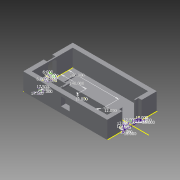
# Autodesk Inventor part: West_Structure_1st_Floor
Saved by Autodesk Inventor 2014 (Build 180170000, 170)
## iProperties
Created: 2013-07-10
Part Number: West_Structure_1st_Floor
Material: Generic
Document SubType Name: Modeling
Designer: jmw3
Density: 1 g/cm^3
Appearance: Default
Author: jmw3
Autodesk Inventor part; units mm, degrees
ref_plane "YZ Plane" through (0, 0, 0) normal (1, 0, 0) x (0, 1, 0)
ref_plane "XZ Plane" through (0, 0, 0) normal (0, 1, 0) x (-1, 0, 0)
ref_plane "XY Plane" through (0, 0, 0) normal (0, 0, 1) x (1, 0, 0)
sketch "Sketch1" plane through (0, 0, 0) normal (0, 0, 1) x (1, 0, 0)
  line L0 (-8321.04, 0) -> (8321.04, 0) projected
  line L1 (-5943.6, 3505.2) -> (5943.6, 3505.2)
  line L2 (-5334, 2895.6) -> (5334, 2895.6)
  line L3 (-4572, 2895.6) -> (-4419.6, 2895.6)
  line L4 (-1981.2, -2006.6) -> (-4445, -2006.6)
  line L5 (-4445, -2006.6) -> (-4445, -1892.3)
  line L6 (-1219.2, -2895.6) -> (-1066.8, -2895.6)
  line L7 (5334, -2895.6) -> (0, -2895.6)
  line L8 (0, -2895.6) -> (-5334, -2895.6)
  line L9 (5943.6, -3505.2) -> (0, -3505.2)
  line L10 (0, -3505.2) -> (-5943.6, -3505.2)
  line L11 (5334, 914.4) -> (5943.6, 914.4)
  line L12 (5943.6, -914.4) -> (5334, -914.4)
  line L13 (5334, 2895.6) -> (5334, 914.4)
  line L14 (5334, -914.4) -> (5334, -2895.6)
  line L15 (5943.6, 3505.2) -> (5943.6, 914.4)
  line L16 (5943.6, -914.4) -> (5943.6, -3505.2)
  line L17 (-4445, -2006.6) -> (5334, -2006.6)
  line L18 (5334, -1892.3) -> (-4445, -1892.3)
  line L19 (-4445, -1892.3) -> (-4445, -2006.6)
  line L20 (5334, -1892.3) -> (5334, -2006.6)
  line L21 (-5943.6, 609.6) -> (-5334, 609.6)
  line L22 (-5334, -609.6) -> (-5943.6, -609.6)
  line L23 (-5943.6, -3505.2) -> (-5943.6, -609.6)
  line L24 (-5943.6, 609.6) -> (-5943.6, 3505.2)
  line L25 (-5334, -2895.6) -> (-5334, -609.6)
  line L26 (-5334, 609.6) -> (-5334, 2895.6)
  line L27 (-4445, -2006.6) -> (-4419.6, -2006.6)
  line L28 (-4419.6, 2895.6) -> (-4572, 2895.6)
  line L29 (-4445, -1892.3) -> (-4445, -2006.6)
  line L30 (0, -4907.28) -> (0, 4907.28) projected
  dimension "d202" = 0
  dimension "d18" = 7010.4
  dimension "d19" = 609.6
  dimension "d20" = 609.6
  dimension "d23" = 1828.8
  dimension "d24" = 2590.8
  dimension "d25" = 609.6
  dimension "d28" = 114.3
  dimension "d29" = 0
  dimension "d34" = 1219.2
  dimension "d35" = 2895.6
  dimension "d36" = 609.6
  dimension "d46" = 889
  dimension "d105" = 889
  dimension "d106" = 11887.2
  constraints: 58 end point, 17 parallel, 8 horizontal, 7 collinear, 6 perpendicular, 4 point on line, 2 other
  measures "d18" distance between parallel lines of L10 L1
  measures "d19" distance between parallel lines of L10 L8
  measures "d20" distance between parallel lines of L1 L2
  measures "d23" distance between parallel lines of L12 L11
  measures "d24" distance between parallel lines of L9 L12
  measures "d25" distance between parallel lines of L15 L13
  measures "d28" distance between parallel lines of L17 L18
  measures "d29" distance between parallel lines of L13 L20
  measures "d34" distance between parallel lines of L22 L21
  measures "d35" distance between parallel lines of L10 L22
  measures "d36" distance between parallel lines of L24 L26
  measures "d46" distance between parallel lines of L26 L5
  measures "d105" distance from line of L6.end L17
  measures "d106" distance between parallel lines of L15 L24
extrude "Extrusion9" add sketch "Sketch1" along normal blind 2438.4 contours L18 L14 L17 L30 | L30 L17 L4 L5 L18 | L1 L30 L2 L26 L21 L24 | L1 L15 L11 L13 L2 L30 | L14 L12 L16 L9 L30 L7 | L30 L10 L23 L22 L25 L8 L6
sketch "Sketch8" plane through (0, 0, 0) normal (0, 0, -1) x (-1, 0, 0)
  line L0 (5943.6, 3505.2) -> (-5943.6, 3505.2) projected
  line L1 (-5943.6, 3505.2) -> (-5943.6, 914.4) projected
  line L2 (-5943.6, 914.4) -> (-5334, 914.4) projected
  line L3 (-5334, 914.4) -> (-5334, 2895.6) projected
  line L4 (-5334, 2895.6) -> (5334, 2895.6) projected
  line L5 (5334, 2895.6) -> (5334, 609.6) projected
  line L6 (5334, 609.6) -> (5943.6, 609.6) projected
  line L7 (5943.6, 609.6) -> (5943.6, 3505.2) projected
  line L8 (-5943.6, 3505.2) -> (5943.6, 3505.2)
  line L9 (5943.6, 3505.2) -> (5943.6, -3505.2)
  line L10 (5943.6, -3505.2) -> (-5943.6, -3505.2)
  line L11 (-5943.6, -3505.2) -> (-5943.6, 3505.2)
  point P0 (0, 0)
  constraints: 8 end point, 2 parallel, 1 horizontal, 1 perpendicular
extrude "Extrusion10" add sketch "Sketch8" along normal blind 25.4
sketch "Sketch9" plane through (0, 0, 2438.4) normal (0, 0, 1) x (1, 0, 0)
  line L0 (5943.6, 3505.2) -> (-5943.6, 3505.2) projected
  line L1 (-5943.6, 3505.2) -> (-5943.6, 609.6) projected
  line L2 (-5943.6, 609.6) -> (-5334, 609.6) projected
  line L3 (-5334, 609.6) -> (-5334, 2895.6) projected
  line L4 (-5334, 2895.6) -> (5334, 2895.6) projected
  line L5 (5334, 2895.6) -> (5334, 914.4) projected
  line L6 (5334, 914.4) -> (5943.6, 914.4) projected
  line L7 (5943.6, 914.4) -> (5943.6, 3505.2) projected
  line L8 (-5943.6, 609.6) -> (-5334, 609.6)
  line L9 (-5334, 609.6) -> (-5334, -609.6)
  line L10 (-5334, -609.6) -> (-5943.6, -609.6)
  line L11 (-5943.6, -609.6) -> (-5943.6, 609.6)
  line L12 (5334, 914.4) -> (5943.6, 914.4)
  line L13 (5943.6, 914.4) -> (5943.6, -914.4)
  line L14 (5943.6, -914.4) -> (5334, -914.4)
  line L15 (5334, -914.4) -> (5334, 914.4)
  point P0 (0, 0)
  constraints: 16 end point, 4 parallel, 2 horizontal, 2 perpendicular
extrude "Extrusion11" add sketch "Sketch9" against normal blind 406.4 contours L13 L14 L15 L6 | L2 L9 L10 L11
sketch "Sketch10" plane through (-4445, -2006.6, 2438.4) normal (0, -1, 0) x (1, 0, 0)
  line L0 (0, -2438.4) -> (9779, -2438.4) projected
  line L1 (0, -2438.4) -> (0, 0) projected
  line L2 (723.9, -2438.4) -> (914.4, -2438.4)
  line L3 (914.4, -2438.4) -> (914.4, -2254.25)
  line L4 (914.4, -2254.25) -> (723.9, -2254.25)
  line L5 (723.9, -2254.25) -> (723.9, -2438.4)
  line L6 (914.4, -2254.25) -> (1104.9, -2254.25)
  line L7 (1104.9, -2254.25) -> (1104.9, -2070.1)
  line L8 (1104.9, -2070.1) -> (914.4, -2070.1)
  line L9 (914.4, -2070.1) -> (914.4, -2254.25)
  line L10 (1104.9, -2070.1) -> (1295.4, -2070.1)
  line L11 (1295.4, -2070.1) -> (1295.4, -1885.95)
  line L12 (1295.4, -1885.95) -> (1104.9, -1885.95)
  line L13 (1104.9, -1885.95) -> (1104.9, -2070.1)
  line L14 (1295.4, -1885.95) -> (1485.9, -1885.95)
  line L15 (1485.9, -1885.95) -> (1485.9, -1701.8)
  line L16 (1485.9, -1701.8) -> (1295.4, -1701.8)
  line L17 (1295.4, -1701.8) -> (1295.4, -1885.95)
  line L18 (1485.9, -1701.8) -> (1676.4, -1701.8)
  line L19 (1676.4, -1701.8) -> (1676.4, -1517.65)
  line L20 (1676.4, -1517.65) -> (1485.9, -1517.65)
  line L21 (1485.9, -1517.65) -> (1485.9, -1701.8)
  line L22 (1676.4, -1517.65) -> (1866.9, -1517.65)
  line L23 (1866.9, -1517.65) -> (1866.9, -1333.5)
  line L24 (1866.9, -1333.5) -> (1676.4, -1333.5)
  line L25 (1676.4, -1333.5) -> (1676.4, -1517.65)
  line L26 (1866.9, -1333.5) -> (2057.4, -1333.5)
  line L27 (2057.4, -1333.5) -> (2057.4, -1149.35)
  line L28 (2057.4, -1149.35) -> (1866.9, -1149.35)
  line L29 (1866.9, -1149.35) -> (1866.9, -1333.5)
  line L30 (2438.4, -965.2) -> (2438.4, -781.05)
  line L31 (2247.9, -1149.35) -> (2247.9, -965.2)
  line L32 (2247.9, -965.2) -> (2438.4, -965.2)
  line L33 (2438.4, -781.05) -> (2247.9, -781.05)
  line L34 (2247.9, -781.05) -> (2247.9, -965.2)
  line L35 (2057.4, -1149.35) -> (2247.9, -1149.35)
  line L36 (2247.9, -965.2) -> (2057.4, -965.2)
  line L37 (2057.4, -965.2) -> (2057.4, -1149.35)
  line L38 (2628.9, -781.05) -> (2628.9, -596.9)
  line L39 (2438.4, -781.05) -> (2628.9, -781.05)
  line L40 (2628.9, -596.9) -> (2438.4, -596.9)
  line L41 (2438.4, -596.9) -> (2438.4, -781.05)
  line L42 (3200.4, -228.6) -> (3200.4, -44.45)
  line L43 (3200.4, 139.7) -> (3200.4, -44.45)
  line L44 (3200.4, -44.45) -> (3390.9, -44.45)
  line L45 (3390.9, 139.7) -> (3200.4, 139.7)
  line L46 (3009.9, -44.45) -> (3009.9, -228.6)
  line L47 (3009.9, -228.6) -> (3200.4, -228.6)
  line L48 (3200.4, -44.45) -> (3009.9, -44.45)
  line L49 (3390.9, -44.45) -> (3390.9, 139.7)
  line L50 (3009.9, -412.75) -> (3009.9, -228.6)
  line L51 (3009.9, -228.6) -> (2819.4, -228.6)
  line L52 (2819.4, -412.75) -> (3009.9, -412.75)
  line L53 (2819.4, -228.6) -> (2819.4, -412.75)
  line L54 (2819.4, -596.9) -> (2819.4, -412.75)
  line L55 (2819.4, -412.75) -> (2628.9, -412.75)
  line L56 (2628.9, -596.9) -> (2819.4, -596.9)
  line L57 (2628.9, -412.75) -> (2628.9, -596.9)
  line L58 (3390.9, 139.7) -> (3581.4, 139.7)
  line L59 (3581.4, 139.7) -> (3581.4, 323.85)
  line L60 (3581.4, 323.85) -> (3390.9, 323.85)
  line L61 (3390.9, 323.85) -> (3390.9, 139.7)
  point P0 (8445.5, -2438.4)
  point P1 (4445, -2438.4)
  dimension "d113" = 190.5
  dimension "d115" = 184.15
  dimension "d116" = 723.9
  dimension "d117" = 190.5
  dimension "d118" = 184.15
  dimension "d119" = 190.5
  dimension "d120" = 184.15
  dimension "d121" = 190.5
  dimension "d122" = 184.15
  dimension "d123" = 190.5
  dimension "d124" = 184.15
  dimension "d125" = 190.5
  dimension "d126" = 184.15
  dimension "d127" = 190.5
  dimension "d128" = 184.15
  dimension "d129" = 190.5
  dimension "d130" = 184.15
  dimension "d131" = 190.5
  dimension "d132" = 184.15
  dimension "d133" = 190.5
  dimension "d134" = 184.15
  dimension "d135" = 190.5
  dimension "d136" = 184.15
  dimension "d137" = 190.5
  dimension "d138" = 184.15
  dimension "d139" = 190.5
  dimension "d140" = 184.15
  dimension "d141" = 190.5
  dimension "d142" = 184.15
  dimension "d154" = 184.15
  dimension "d155" = 190.5
  constraints: 120 end point, 30 parallel, 15 horizontal, 15 perpendicular, 12 collinear, 1 point on line
  measures "d113" distance between parallel lines of L3 L5
  measures "d115" distance between parallel lines of L4 L0
  measures "d116" distance between parallel lines of L1 L5
  measures "d117" distance between parallel lines of L9 L7
  measures "d118" distance between parallel lines of L8 L6
  measures "d119" distance between parallel lines of L11 L13
  measures "d120" distance between parallel lines of L12 L10
  measures "d121" distance between parallel lines of L17 L15
  measures "d122" distance between parallel lines of L16 L14
  measures "d123" distance between parallel lines of L19 L21
  measures "d124" distance between parallel lines of L20 L18
  measures "d125" distance between parallel lines of L25 L23
  measures "d126" distance between parallel lines of L24 L22
  measures "d127" distance between parallel lines of L27 L29
  measures "d128" distance between parallel lines of L28 L26
  measures "d129" distance between parallel lines of L37 L31
  measures "d130" distance between parallel lines of L36 L35
  measures "d131" distance between parallel lines of L30 L34
  measures "d132" distance between parallel lines of L33 L32
  measures "d133" distance between parallel lines of L38 L41
  measures "d134" distance between parallel lines of L40 L39
  measures "d135" distance between parallel lines of L57 L54
  measures "d136" distance between parallel lines of L55 L56
  measures "d137" distance between parallel lines of L50 L53
  measures "d138" distance between parallel lines of L51 L52
  measures "d139" distance between parallel lines of L46 L42
  measures "d140" distance between parallel lines of L48 L47
  measures "d141" distance between parallel lines of L49 L43
  measures "d142" distance between parallel lines of L45 L44
  measures "d154" distance between parallel lines of L58 L60
  measures "d155" distance between parallel lines of L61 L59
extrude "Extrusion12" add sketch "Sketch10" along normal up to surface (889 mm away)
sketch "Sketch11" plane through (-5943.6, -3505.2, 2438.4) normal (0, -1, 0) x (1, 0, 0)
  line L0 (5334, -406.4) -> (6553.2, -406.4)
  line L1 (6553.2, -406.4) -> (6553.2, -1625.6)
  line L2 (6553.2, -1625.6) -> (5334, -1625.6)
  line L3 (5334, -1625.6) -> (5334, -406.4)
  line L4 (11277.6, -2438.4) -> (2413, -2438.4) projected
  line L5 (5943.6, -2956.56) -> (5943.6, 492.76) projected
  point P0 (5943.6, -2438.4)
  dimension "d145" = 1219.2
  dimension "d147" = 1219.2
  dimension "d148" = 812.8
  constraints: 8 end point, 2 parallel, 1 horizontal, 1 perpendicular, 1 other
  measures "d145" distance between parallel lines of L0 L2
  measures "d147" distance between parallel lines of L1 L3
  measures "d148" distance between parallel lines of L4 L2
extrude "Extrusion13" cut sketch "Sketch11" against normal up to surface (609.6 mm away)
sketch "Sketch14" plane through (0, 0, 2032) normal (0, 0, -1) x (-1, 0, 0)
  line L0 (-5334, -914.4) -> (-5334, 914.4) projected
  line L1 (-5943.6, 914.4) -> (-5943.6, -914.4) projected
  line L2 (-8321.04, 0) -> (8321.04, 0) projected
  line L3 (-5943.6, 12.7) -> (-5334, 12.7)
  line L4 (-5334, 12.7) -> (-5334, -12.7)
  line L5 (-5334, -12.7) -> (-5943.6, -12.7)
  line L6 (-5943.6, -12.7) -> (-5943.6, 12.7)
  point P0 (0, 0)
  dimension "d156" = 25.4
  constraints: 8 end point, 2 parallel, 2 point on line, 1 horizontal, 1 perpendicular, 1 other
  measures "d156" distance between parallel lines of L3 L5
extrude "Extrusion15" add sketch "Sketch14" along normal blind 25.4
sketch "Sketch15" plane through (0, 0, 0) normal (0, 0, 1) x (1, 0, 0)
  line L0 (5334, -914.4) -> (5334, -1892.3) projected
  line L1 (5943.6, -914.4) -> (5334, -914.4) projected
  line L2 (5943.6, 914.4) -> (5334, 914.4) projected
  line L3 (5334, 914.4) -> (5334, 2895.6) projected
  line L4 (-5334, 2895.6) -> (-5334, 609.6) projected
  line L5 (-5334, -609.6) -> (-5943.6, -609.6) projected
  line L6 (-3721.1, -2895.6) -> (-5334, -2895.6) projected
  line L7 (-8321.04, 0) -> (8321.04, 0) projected
  circle A0 centre (1778, 0) radius 152.4
  line L8 (-4445, -2006.6) -> (-5334, -2006.6)
  line L9 (-5334, -2006.6) -> (-5334, -2895.6)
  line L10 (-5334, -2895.6) -> (-4445, -2895.6)
  line L11 (-4445, -2895.6) -> (-4445, -2006.6)
  circle A1 centre (-4889.5, -2451.1) radius 152.4
  line L12 (-5181.6, -152.4) -> (-5486.4, -152.4)
  line L13 (-5486.4, -152.4) -> (-5486.4, 152.4)
  line L14 (-5486.4, 152.4) -> (-5181.6, -152.4)
  line L15 (5486.4, 304.8) -> (5181.6, 304.8)
  line L16 (5181.6, 304.8) -> (5181.6, 609.6)
  line L17 (5181.6, 609.6) -> (5486.4, 304.8)
  line L18 (5486.4, -609.6) -> (5181.6, -609.6)
  line L19 (5181.6, -304.8) -> (5486.4, -609.6)
  line L20 (5181.6, -609.6) -> (5181.6, -304.8)
  line L21 (-5943.6, -3505.2) -> (-5943.6, 3505.2) projected
  line L22 (-5334, -609.6) -> (-5943.6, -609.6)
  line L23 (-5943.6, -609.6) -> (-5943.6, 609.6)
  line L24 (-5943.6, 609.6) -> (-5334, 609.6)
  line L25 (-5334, 609.6) -> (-5334, -609.6)
  line L26 (-5486.4, 609.6) -> (-5334, 609.6)
  line L27 (-5334, 609.6) -> (-5334, 457.2)
  line L28 (-5334, 457.2) -> (-5486.4, 457.2)
  line L29 (-5486.4, 457.2) -> (-5486.4, 609.6)
  line L30 (-5334, -609.6) -> (-5486.4, -609.6)
  line L31 (-5486.4, -609.6) -> (-5486.4, -457.2)
  line L32 (-5486.4, -457.2) -> (-5334, -457.2)
  line L33 (-5334, -457.2) -> (-5334, -609.6)
  line L34 (5943.6, 3505.2) -> (5943.6, -3505.2) projected
  line L35 (5486.4, 914.4) -> (5943.6, 914.4)
  line L36 (5943.6, 914.4) -> (5943.6, 1371.6)
  line L37 (5943.6, 1371.6) -> (5486.4, 1371.6)
  line L38 (5486.4, 1371.6) -> (5486.4, 914.4)
  line L39 (5943.6, -914.4) -> (5486.4, -914.4)
  line L40 (5486.4, -914.4) -> (5486.4, -1371.6)
  line L41 (5486.4, -1371.6) -> (5943.6, -1371.6)
  line L42 (5943.6, -1371.6) -> (5943.6, -914.4)
  line L43 (5486.4, 914.4) -> (6132.9784, 1560.9784)
  line L44 (6132.9784, 1560.9784) -> (6240.7415, 1453.2154)
  line L45 (6240.7415, 1453.2154) -> (5594.1631, 806.6369)
  line L46 (5486.4, 914.4) -> (5594.1631, 806.6369)
  line L47 (5486.4, -914.4) -> (6132.9784, -1560.9784)
  line L48 (6132.9784, -1560.9784) -> (6240.7415, -1453.2154)
  line L49 (6240.7415, -1453.2154) -> (5594.1631, -806.6369)
  line L50 (5486.4, -914.4) -> (5594.1631, -806.6369)
  line L51 (5486.4, 1371.6) -> (5943.6, 1371.6)
  line L52 (5943.6, 1371.6) -> (5943.6, -1371.6)
  line L53 (5943.6, -1371.6) -> (5486.4, -1371.6)
  line L54 (5486.4, -1371.6) -> (5486.4, 1371.6)
  line L55 (-5486.4, 457.2) -> (-6353.876, 746.3587)
  line L56 (-6353.876, 746.3587) -> (-6402.0691, 601.7793)
  line L57 (-6402.0691, 601.7793) -> (-5534.5931, 312.6207)
  line L58 (-5486.4, 457.2) -> (-5534.5931, 312.6207)
  line L59 (5334, 914.4) -> (5486.4, 914.4)
  line L60 (5486.4, 914.4) -> (5486.4, 0)
  line L61 (5486.4, 0) -> (5334, 0)
  line L62 (5334, 0) -> (5334, 914.4)
  line L63 (-4889.5, -2451.1) -> (-5041.9, -2363.1118)
  line L64 (-5041.9, -2363.1118) -> (-5041.9, -2187.1355)
  line L65 (-5041.9, -2187.1355) -> (-4889.5, -2099.1473)
  line L66 (-4889.5, -2099.1473) -> (-4737.1, -2187.1355)
  line L67 (-4737.1, -2187.1355) -> (-4737.1, -2363.1118)
  line L68 (-4737.1, -2363.1118) -> (-4889.5, -2451.1)
  circle A2 centre (-1778, 0) radius 152.4
  point P0 (0, 0)
  point P1 (-5334, 0)
  point P2 (1.5875, 1.5875)
  point P3 (770.0638, -2405.9824)
  point P4 (-4729.4618, 0)
  point P5 (5334, 457.2)
  point P6 (5334, -457.2)
  point P7 (-4889.5, -2275.1236)
  dimension "d161" = 304.8
  dimension "d165" = 7112
  dimension "d166" = 304.8
  dimension "d167" = 444.5
  dimension "d172" = 304.8
  dimension "d173" = 304.8
  dimension "d174" = 152.4
  dimension "d176" = 304.8
  dimension "d177" = 304.8
  dimension "d180" = 304.8
  dimension "d181" = 304.8
  dimension "d184" = 457.2
  dimension "d192" = 152.4
  dimension "d193" = 152.4
  dimension "d194" = 152.4
  dimension "d195" = 457.2
  dimension "d196" = 457.2
  dimension "d197" = 457.2
  dimension "d198" = 457.2
  dimension "d199" = 914.4
  dimension "d200" = 152.4
  dimension "d215" = 152.4
  dimension "d216" = 914.4
  dimension "d231" = 304.8
  dimension "d232" = 444.5
  dimension "d237" = 304.8
  dimension "d238" = 3556
  constraints: 118 end point, 23 parallel, 14 perpendicular, 12 point on line, 8 horizontal, 4 midpoint, 3 centre point, 3 symmetric about line, 1 coincident, 1 collinear, 13 other
  measures "d161" diameter of A0
  measures "d165" distance from line of L4 A0.centre
  measures "d166" diameter of A1
  measures "d167" distance from line of L6 A1.centre
  measures "d172" distance of L12.start L12.end
  measures "d173" distance of L12.end L13.end
  measures "d174" distance from line of point (-5334, 0) L13
  measures "d176" distance of L15.start L15.end
  measures "d177" distance of L15.end L17.start
  measures "d180" distance of L19.end L20.start
  measures "d181" distance of L20.start L20.end
  measures "d184" distance from line of L1 point (5334, -457.2)
  measures "d192" distance between parallel lines of L27 L29
  measures "d193" distance between parallel lines of L26 L28
  measures "d194" distance between parallel lines of L5 L32
  measures "d195" distance between parallel lines of L35 L37
  measures "d196" distance between parallel lines of L38 L34
  measures "d197" distance between parallel lines of L40 L42
  measures "d198" distance between parallel lines of L1 L41
  measures "d199" distance between parallel lines of L44 L46
  measures "d200" distance between parallel lines of L43 L45
  measures "d215" distance between parallel lines of L57 L55
  measures "d216" distance between parallel lines of L58 L56
  measures "d231" distance between parallel lines of L64 L67
  measures "d232" distance from line of L9 A1.centre
  measures "d237" diameter of A2
  measures "d238" distance from line of L4 A2.centre
extrude "Extrusion18" add sketch "Sketch15" along normal blind 25.4 contours L18 L20 L19 | L15 L62 L17 | L15 L16 L17 L62
extrude "Extrusion19" cut sketch "Sketch15" along normal up to surface (2438.4 mm away) contours L34 L49 L1 | L1 L49 L50 L54 L7 L34 | L49 L34 L47 L1 | L1 L50 L49 | L7 L54 L46 L45 L2 L34 | L47 L41 L40 | L2 L45 L34 | L45 L46 L2 | L2 L43 L34 L45 | L38 L37 L43
extrude "Extrusion20" add sketch "Sketch15" along normal blind 25.4 contours L18 L20 L19 | L15 L62 L17 | L15 L16 L17 L62
sketch "Sketch16" plane through (0, 0, 2438.4) normal (0, 0, 1) x (1, 0, 0)
  line L0 (5486.4, 914.4) -> (5334, 914.4) projected
  line L1 (5334, -914.4) -> (5486.4, -914.4) projected
  line L2 (5334, 914.4) -> (5486.4, 914.4)
  line L3 (5486.4, 914.4) -> (5486.4, -914.4)
  line L4 (5486.4, -914.4) -> (5334, -914.4)
  line L5 (5334, -914.4) -> (5334, 914.4)
  point P0 (0, 0)
  constraints: 8 end point, 2 parallel, 1 horizontal, 1 perpendicular
extrude "Extrusion22" cut sketch "Sketch16" against normal up to surface (431.8 mm away)
sketch "Sketch17" plane through (0, 0, 2438.4) normal (0, 0, 1) x (1, 0, 0)
  line L0 (-5334, -2895.6) -> (-5334, 2895.6) projected
  line L1 (-5943.6, 3505.2) -> (-5943.6, -3505.2) projected
  line L2 (-5334, 609.6) -> (-5334, -609.6) projected
  line L3 (-5486.4, 457.2) -> (-5486.4, 609.6) projected
  line L4 (-5334, 457.2) -> (-5486.4, 457.2) projected
  line L5 (-5334, 609.6) -> (-5943.6, 609.6) projected
  line L6 (-5486.4, -457.2) -> (-5334, -457.2) projected
  line L7 (-5486.4, -609.6) -> (-5486.4, -457.2) projected
  line L8 (-5334, -609.6) -> (-5943.6, -609.6) projected
  point P0 (0, 0)
extrude "Extrusion23" cut sketch "Sketch17" against normal up to surface (406.4 mm away) contours L6 L7 L8 L1 L5 L3 L4 L0
sketch "Sketch18" plane through (-5486.4, 457.2, 2438.4) normal (0, -1, 0) x (1, 0, 0)
  line L0 (152.4, 0) -> (152.4, -406.4) projected
  line L1 (0, 0) -> (152.4, 0)
  line L2 (152.4, 0) -> (152.4, -203.2)
  line L3 (152.4, -203.2) -> (0, -203.2)
  line L4 (0, -203.2) -> (0, 0)
  point P0 (5486.4, -2438.4)
  constraints: 8 end point, 2 parallel, 1 horizontal, 1 midpoint, 1 perpendicular
extrude "Extrusion24" add sketch "Sketch18" along normal up to surface (914.4 mm away)
extrude "Extrusion25" cut sketch "Sketch15" along normal blind 25.4 contours L18 L20 L19 | L15 L62 L17 | L15 L16 L17 L62
extrude "Extrusion28" add sketch "Sketch15" along normal blind 25.4 contours L7 L62 L15 L54 | L15 L62 L17 | L17 L62 L2 L54
extrude "Extrusion29" cut sketch "Sketch15" against normal blind 25.4 contours L34 L49 L1 | L1 L49 L50 L54 L7 L34 | L49 L34 L47 L1 | L1 L50 L49 | L7 L54 L46 L45 L2 L34 | L47 L41 L40 | L2 L45 L34 | L45 L46 L2 | L2 L43 L34 L45 | L38 L37 L43
extrude "Extrusion30" cut sketch "Sketch15" against normal blind 25.4 contours L25 L12 L13 L7 | L7 L13 L14 | L14 L13 L7 L21 L57 L58 L28 L25 | L13 L12 L25 L32 L31 L5 L21 L7 | L28 L29 L24 L25 | L58 L57 L21 L55 | L25 L5 L31 L32
sketch "Sketch20" plane through (0, 0, 0) normal (0, 0, 1) x (1, 0, 0)
  line L0 (5334, 2895.6) -> (-5334, 2895.6) projected
  line L1 (-5334, 2895.6) -> (-5334, 609.6) projected
  line L2 (-4724.4, 2286) -> (-4060.825, 2286)
  line L3 (-4060.825, 2286) -> (-4060.825, 295.275)
  line L4 (-4060.825, 295.275) -> (-4724.4, 295.275)
  line L5 (-4724.4, 295.275) -> (-4724.4, 2286)
  point P0 (0, 0)
  dimension "d227" = 1990.725
  dimension "d228" = 663.575
  dimension "d229" = 609.6
  dimension "d230" = 609.6
  constraints: 8 end point, 2 parallel, 1 horizontal, 1 perpendicular
  measures "d227" distance between parallel lines of L2 L4
  measures "d228" distance between parallel lines of L3 L5
  measures "d229" distance between parallel lines of L0 L2
  measures "d230" distance between parallel lines of L1 L5
extrude "Extrusion31" add sketch "Sketch15" along normal blind 25.4 contours L18 L20 L19 | L14 L12 L25 | L25 L12 L13 L7 | L7 L13 L14 | L15 L62 L17 | L15 L16 L17 L62 | A1 L63 L68 | L68 L63 A1 | A1 L63 L64 L65 L66 L67 L68
extrude "Burners" add sketch "Sketch20" along normal blind 139.7
sketch "Sketch12" plane through (0, 0, 2438.4) normal (0, 0, 1) x (1, 0, 0)
  line L0 (-5943.6, -3505.2) -> (5943.6, -3505.2) projected
  line L1 (5943.6, -3505.2) -> (5943.6, 3505.2) projected
  line L2 (5943.6, 3505.2) -> (-5943.6, 3505.2) projected
  line L3 (-5943.6, 3505.2) -> (5943.6, 3505.2)
  line L4 (5943.6, 3505.2) -> (5943.6, -2463.8)
  line L5 (5943.6, -2463.8) -> (-5943.6, -2463.8)
  line L6 (-5943.6, -2463.8) -> (-5943.6, 3505.2)
  line L7 (-1054.1, -2006.6) -> (5943.6, -2006.6)
  line L8 (5943.6, -2006.6) -> (5943.6, -3505.2)
  line L9 (5943.6, -3505.2) -> (-1054.1, -3505.2)
  line L10 (-1054.1, -3505.2) -> (-1054.1, -2006.6)
  line L11 (-5943.6, -2463.8) -> (-5181.6, -2463.8)
  line L12 (-5181.6, -2463.8) -> (-5181.6, -3505.2)
  line L13 (-5181.6, -3505.2) -> (-5943.6, -3505.2)
  line L14 (-5943.6, -3505.2) -> (-5943.6, -2463.8)
  line L15 (-1054.1, -2895.6) -> (-5943.6, -2895.6)
  line L16 (-5943.6, -2895.6) -> (-5943.6, -3505.2)
  line L17 (-5943.6, -3505.2) -> (-1054.1, -3505.2)
  line L18 (-1054.1, -3505.2) -> (-1054.1, -2895.6)
  point P0 (0, 0)
  constraints: 32 end point, 8 parallel, 4 horizontal, 4 perpendicular, 2 point on line
body "Solid2"
